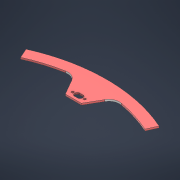
# Autodesk Inventor part: sensor
Saved by Autodesk Inventor 2022 (Build 260153000, 153)
## iProperties
Created: 2021-10-17
Part Number: sensor
Material: 一般
Document SubType Name: Modeling
Designer: shiok
Density: 1 g/cm^3
Appearance: 既定
Author: shiok
Autodesk Inventor part; units mm, degrees
ref_plane "YZ Plane" through (0, 0, 0) normal (1, 0, 0) x (0, 1, 0)
ref_plane "XZ Plane" through (0, 0, 0) normal (0, 1, 0) x (-1, 0, 0)
ref_plane "XY Plane" through (0, 0, 0) normal (0, 0, 1) x (1, 0, 0)
sketch "スケッチ1" plane through (0, 0, 0) normal (0, 1, 0) x (-1, 0, 0)
  arc A0 (0, -153.7673) -> (62.5, -140.4925) centre (0, 0) ccw
  line L0 (62.5, -140.4925) -> (0, 0)
  line L1 (0, 0) -> (0, -153.7673)
  arc A1 (19.047, -142.5) -> (58.4354, -131.3558) centre (0, 0) ccw
  line L2 (19.047, -142.5) -> (7.5, -122.5)
  line L3 (7.5, -122.5) -> (0, -122.5)
  arc A2 (-62.5, -140.4925) -> (0, -153.7673) centre (0, 0) ccw
  line L4 (-62.5, -140.4925) -> (0, 0)
  arc A3 (-58.4354, -131.3558) -> (-19.047, -142.5) centre (0, 0) ccw
  line L5 (-19.047, -142.5) -> (-7.5, -122.5)
  line L6 (-7.5, -122.5) -> (0, -122.5)
  line L7 (19.047, -142.5) -> (0, -142.5) construction
  line L8 (-19.047, -142.5) -> (0, -142.5) construction
  line L9 (0, -130) -> (1.75, -130)
  line L10 (3.75, -128) -> (3.75, -127)
  line L11 (1.75, -125) -> (0, -125)
  arc A4 (3.75, -127) -> (1.75, -125) centre (1.75, -127) ccw
  arc A5 (1.75, -130) -> (3.75, -128) centre (1.75, -128) ccw
  line L12 (0, -130) -> (-1.75, -130)
  line L13 (-3.75, -128) -> (-3.75, -127)
  line L14 (-1.75, -125) -> (0, -125)
  arc A6 (-1.75, -125) -> (-3.75, -127) centre (-1.75, -127) ccw
  arc A7 (-3.75, -128) -> (-1.75, -130) centre (-1.75, -128) ccw
  point P0 (3.75, -130)
  point P1 (3.75, -125)
  dimension "d4" = 15
  dimension "d6" = 60
  dimension "d7" = 20
  dimension "d8" = 125
  dimension "d9" = 2.5
  dimension "d10" = 5
  dimension "d12" = 122.5
  dimension "d13" = 10
  dimension "d14" = 2
  dimension "d16" = 7.5
  constraints: 30 end point, 16 point on circle, 10 point on line, 10 symmetric about line, 8 centre point, 4 coincident, 4 perpendicular, 4 tangent, 1 equal radius, 1 horizontal, 1 vertical, 4 other
  measures "d4" distance of L2.end L5.end
  measures "d6" angle of L2 L3
  measures "d7" distance between parallel lines of L7 L3
  measures "d8" distance of L4.start L0.start
  measures "d9" distance between parallel lines of L11 L3
  measures "d10" distance between parallel lines of L9 L11
  measures "d12" distance from line of point (0, 0) L3
  measures "d13" radial gap between concentric circles of A0 A1
  measures "d14" radius of A4
  measures "d16" distance between parallel lines of L13 L10
extrude "押し出し1" add sketch "スケッチ1" along normal blind 1.6 contours L1 L9 A5 L10 A4 L11 L3 L2 A1 L0 A0 | A2 L4 A3 L5 L6 L1 L14 A6 L13 A7 L12
sketch "スケッチ2" plane through (0, 1.6, 0) normal (0, 1, 0) x (1, 0, 0)
  line L0 (7.5, 122.5) -> (19.047, 142.5) projected
  arc A0 (58.4354, 131.3558) -> (19.047, 142.5) centre (0, 0) ccw projected
  line L1 (58.4354, 131.3558) -> (62.5, 140.4925) projected
  arc A1 (62.5, 140.4925) -> (-62.5, 140.4925) centre (0, 0) ccw projected
  line L2 (-62.5, 140.4925) -> (-58.4354, 131.3558) projected
  arc A2 (-19.047, 142.5) -> (-58.4354, 131.3558) centre (0, 0) ccw projected
  line L3 (-19.047, 142.5) -> (-7.5, 122.5) projected
  line L4 (-7.5, 122.5) -> (7.5, 122.5) projected
  line L5 (1.75, 125) -> (-1.75, 125) projected
  arc A3 (-3.75, 127) -> (-1.75, 125) centre (-1.75, 127) ccw projected
  line L6 (-3.75, 127) -> (-3.75, 128) projected
  arc A4 (-1.75, 130) -> (-3.75, 128) centre (-1.75, 128) ccw projected
  line L7 (-1.75, 130) -> (1.75, 130) projected
  arc A5 (3.75, 128) -> (1.75, 130) centre (1.75, 128) ccw projected
  line L8 (3.75, 128) -> (3.75, 127) projected
  arc A6 (1.75, 125) -> (3.75, 127) centre (1.75, 127) ccw projected
  line L9 (-7.5, 122.5) -> (7.5, 122.5)
  line L10 (7.5, 122.5) -> (7.5, 132.5)
  line L11 (7.5, 132.5) -> (-7.5, 132.5)
  line L12 (-7.5, 132.5) -> (-7.5, 122.5)
  line L13 (-5.625, 127.5) -> (-3.75, 127.5) construction
  line L14 (-3.75, 127) -> (-3.75, 128) projected
  line L15 (-5.625, 127.5) -> (-7.5, 127.5) construction
  line L16 (-1.75, 130) -> (1.75, 130) projected
  line L17 (0, 130) -> (0, 125)
  line L18 (1.75, 125) -> (-1.75, 125) projected
  point P0 (5.625, 127.5)
  dimension "d19" = 10
  dimension "d20" = 15
  constraints: 14 end point, 6 midpoint, 2 collinear, 2 parallel, 1 horizontal, 1 horizontal alignment, 1 perpendicular, 1 symmetric about line
  measures "d19" distance of L10.end L9.end
  measures "d20" distance of L10.end L11.end
hole "穴1" at (5.625, 1.6, -127.5) at (-5.625, 1.6, -127.5) direction (0, -1, 0) diameter 2.4 depth 1.6 tip angle 118 clearance for "Countersunk Flat Head Screw ISO 2009/7046" size "M2" standard "ISO"
fillet "フィレット1" radius 10 2 edges at (19.047, 0.8, -142.5) (-19.047, 0.8, -142.5)
